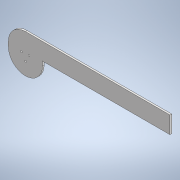
# Autodesk Inventor part: lokiec
Saved by Autodesk Inventor 2022 (Build 260153000, 153)
## iProperties
Created: 2023-01-20
Part Number: lokiec
Material: Generic
Document SubType Name: Modeling
Designer: Kamil
Density: 1 g/cm^3
Appearance: Default
Author: Kamil
Autodesk Inventor part; units mm, degrees
ref_plane "YZ Plane" through (0, 0, 0) normal (1, 0, 0) x (0, 1, 0)
ref_plane "XZ Plane" through (0, 0, 0) normal (0, 1, 0) x (-1, 0, 0)
ref_plane "XY Plane" through (0, 0, 0) normal (0, 0, 1) x (1, 0, 0)
sketch "Sketch1" plane through (0, 0, 0) normal (0, 0, 1) x (1, 0, 0)
  circle A0 centre (0, 0) radius 22.3333 projected
  circle A1 centre (8.5222, 5.6951) radius 2 projected
  circle A2 centre (0.671, -10.228) radius 2 projected
  circle A3 centre (-9.1932, 4.5329) radius 2 projected
  arc A4 (-33.8969, -20.2792) -> (36.2558, -15.6768) centre (0, 0) ccw projected
  arc A5 (39.2843, 4.1223) -> (-39.4862, -1.0454) centre (0, 0) ccw projected
  circle A6 centre (0, 0) radius 39.5
  line L0 (364.1325, 23.8889) -> (45.9013, 3.0114) projected
  line L1 (26.2679, 39.5) -> (334.9329, 39.5)
  line L2 (334.9329, 39.5) -> (334.9329, 0)
  line L3 (39.5, 10) -> (334.9329, 10)
  line L4 (334.9329, 10) -> (334.9329, 0)
  line L5 (334.9329, 39.5) -> (26.2679, 39.5)
  line L6 (0, 49.5) -> (334.9329, 49.5)
  line L7 (334.9329, 49.5) -> (334.9329, 39.5)
  arc A7 (39.1823, 5) -> (26.2679, 39.5) centre (0, 10) ccw
  arc A8 (0, 49.5) -> (-39.1823, 5) centre (0, 10) ccw
  line L8 (0, 0) -> (-39.5, 0)
  line L9 (-39.5, 0) -> (-39.5, 10)
  line L10 (39.5, 0) -> (39.5, 10)
  point P0 (0, 0)
  point P1 (-39.4862, -1.0454)
  point P2 (-33.8969, -20.2792)
  point P3 (36.2558, -15.6768)
  constraints: 20 end point, 11 point on circle, 3 centre point, 3 tangent, 2 horizontal, 1 coincident, 1 concentric, 1 parallel, 1 perpendicular, 1 vertical
extrude "Extrusion1" add sketch "Sketch1" along normal blind 4 contours A0 | A6 A5 A4 | A6 A5 A7 L10 | L9 A8 A5 | A7 L1 L2 L0 L3 | A7 A5 A8 L6 L7 L1 | L0 L2 L3
body "Solid1"
